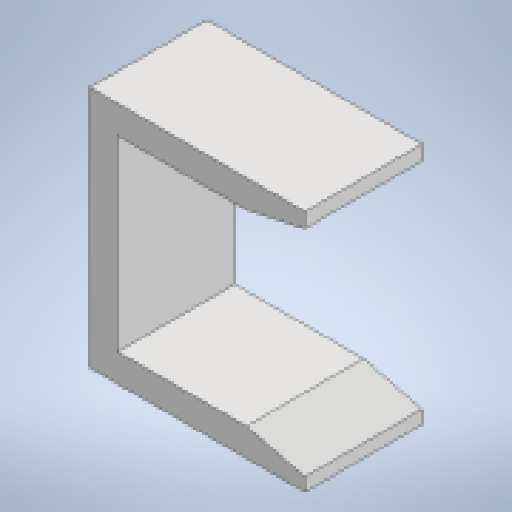
# Autodesk Inventor part: MolexClipper
Saved by Autodesk Inventor 2025.1 (Build 291241000, 241)
## iProperties
Created: 2026-05-09
Part Number: MolexClipper
Material: Generic
Document SubType Name: Modeling
Designer: User
Density: 1 g/cm^3
Appearance: Default
Author: User
## iProperties of the stored document MolexClipper_3DPrint.ipt
Created: 2026-05-09
Part Number: MolexClipper_3DPrint
Material: Generic
Document SubType Name: Modeling
Designer: User
Density: 1 g/cm^3
Appearance: Default
Author: User
Autodesk Inventor part; units mm, degrees
ref_plane "YZ Plane" through (0, 0, 0) normal (1, 0, 0) x (0, 1, 0)
ref_plane "XZ Plane" through (0, 0, 0) normal (0, 1, 0) x (-1, 0, 0)
ref_plane "XY Plane" through (0, 0, 0) normal (0, 0, 1) x (1, 0, 0)
ref_plane "Work Plane1" through (-4.78, -2.9, 8) normal (0, 0, 1) x (1, 0, 0)
sketch "Sketch1" plane through (0, 0, 0) normal (0, 0, 1) x (1, 0, 0)
  line L0 (-6.35, 2.9) -> (-6.35, -2.9)
  line L1 (6.35, 2.9) -> (-6.35, 2.9)
  line L2 (-6.35, -2.9) -> (-5.08, -2.9)
  line L3 (-4.78, -2.9) -> (4.78, -2.9)
  line L4 (-4.78, -2.9) -> (-5.08, -2.9)
  line L5 (5.08, -2.9) -> (6.35, -2.9)
  line L6 (5.08, -2.9) -> (4.78, -2.9)
  line L7 (6.35, 3) -> (-6.45, 3)
  line L8 (-6.45, 3) -> (-6.45, -3)
  line L9 (-6.45, -3) -> (-5.08, -3)
  line L10 (-5.08, -3) -> (-4.78, -3)
  line L11 (-4.78, -3) -> (4.78, -3)
  line L12 (4.78, -3) -> (5.08, -3)
  line L13 (5.08, -3) -> (6.35, -3)
  line L14 (6.35, 4.9) -> (-8.35, 4.9)
  line L15 (-8.35, 4.9) -> (-8.35, -4.9)
  line L16 (-8.35, -4.9) -> (-5.08, -4.9)
  line L17 (-5.08, -4.9) -> (-4.78, -4.9)
  line L18 (-4.78, -4.9) -> (4.78, -4.9)
  line L19 (4.78, -4.9) -> (5.08, -4.9)
  line L20 (5.08, -4.9) -> (6.35, -4.9)
  line L21 (6.35, 4.9) -> (6.35, 3)
  line L22 (6.35, -3) -> (6.35, -4.9)
  line L23 (-6.45, 3) -> (-8.35, 3)
  point P0 (0, 0)
extrude "Extrusion1" add sketch "Sketch1" along normal up to surface (8 mm away) contours L8 L9 L10 L11 L12 L13 L22 L20 L19 L18 L17 L16 L15 L23
chamfer "Chamfer1" distance 1 distance2 4 1 edges at (6.35, -3, 4) measured on face at (6.35, -3.5, 4)
sketch "Sketch2" plane through (-8.35, -4.9, 8) normal (0, 0, 1) x (1, 0, 0)
  line L0 (2, 14.6) -> (2, 8.8)
  line L1 (14.7, 14.6) -> (2, 14.6)
  line L2 (14.7, 14.7) -> (1.9, 14.7)
  line L3 (1.9, 14.7) -> (1.9, 8.8)
  line L4 (0, 8.8) -> (0, 16.6)
  line L5 (0, 16.6) -> (14.7, 16.6)
  line L6 (0, 7.9) -> (1.9, 7.9) projected
  line L7 (1.9, 7.9) -> (1.9, 1.9) projected
  line L8 (1.9, 7.9) -> (1.9, 8.8)
  line L9 (0, 7.9) -> (0, 8.8)
  line L10 (10.7, 1.9) -> (14.7, 0.9) projected
  line L11 (14.7, 16.6) -> (14.7, 15.6)
  line L12 (14.7, 15.6) -> (10.7, 14.7)
  point P0 (8.35, 4.9)
  dimension "d7" = 0.1
  dimension "d8" = 2
  dimension "d9" = 1
  constraints: 20 end point, 2 vertical, 1 horizontal, 1 parallel, 1 point on line, 5 other
  measures "d7" distance between parallel lines of L1 L2
  measures "d8" distance between parallel lines of L0 L4
  measures "d9" distance of L5.end L11.end
extrude "Extrusion2" add sketch "Sketch2" against normal up to surface (8 mm away)
body "Solid1"
